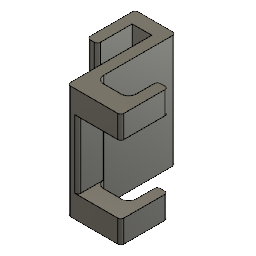
inovativ_combo_mount (Autodesk Fusion 360 design; units mm, degrees)
Autodesk Fusion 360 part; units mm, degrees
sketch "Sketch1" plane through (0, 0, 0) normal (0, 1, 0) x (1, 0, 0)
  line L0 (-10.8509, -30.1905) -> (-10.8509, -7.1905)
  line L1 (-10.8509, -7.1905) -> (2.1491, -7.1905)
  line L2 (2.1491, -7.1905) -> (2.1491, -63.1905)
  line L3 (2.1491, -63.1905) -> (9.1491, -63.1905)
  line L4 (9.1491, -63.1905) -> (9.1491, 1.8095)
  line L5 (9.1491, 1.8095) -> (-17.8509, 1.8095)
  line L6 (-17.8509, 1.8095) -> (-17.8509, -30.1905)
  line L7 (-17.8509, -30.1905) -> (-10.8509, -30.1905)
  line L8 (9.1491, -63.1905) -> (38, -63.1905)
  line L9 (37.6491, -63.1989) -> (37.6491, -32)
  line L10 (37.6491, -32) -> (30.6491, -32)
  line L11 (30.6491, -32) -> (30.6491, -51)
  line L12 (30.6491, -51) -> (9.1491, -51)
  dimension "d11" = 65
  dimension "d15" = 27
  dimension "d16" = 7
  dimension "d17" = 13
  dimension "d18" = 23
  dimension "d24" = 35.5
  dimension "d28" = 21.5
  dimension "d29" = 7
  dimension "d37" = 32
  measures "d24" distance of origin
  measures "d28" distance of origin
extrude "Extrude2" add sketch "Sketch1" along normal blind 75 makes body 1
fillet "Fillet4" radius 5 2 edges at (9.1491, 37.5, 51) (30.6491, 37.5, 51) on bodies 1
box "BoxPrimitive1" add length 45 width 45 height 45 placed x (0, 0, 1) y (1, 0, 0) z (0, 1, 0) at (45, 0, 23) separate body makes body 2
move_body "Move9" bodies 2 to x (1, 0, 0) y (0, 1, 0) z (0, 0, 1) at (-35.8367, 15, -2.9383)
combine "Combine1" operation cut target body 1 tool bodies 2
fillet "Fillet5" radius 2 8 edges at (2.1491, 37.5, 63.1905) (37.6491, 7.5, 63.1905) (37.6491, 67.5, 63.1905) (9.1633, 37.5, 63.1905) (30.6491, 7.5, 32) (37.6491, 7.5, 32) (30.6491, 67.5, 32) (37.6491, 67.5, 32) on bodies 1
fillet "Fillet6" radius 2 4 edges at (-17.8509, 37.5, 30.1905) (9.1491, 37.5, -1.8095) (-17.8509, 37.5, -1.8095) (-10.8509, 37.5, 30.1905) on bodies 1
